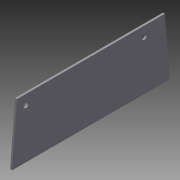
# Autodesk Inventor part: mountPiece
Saved by Autodesk Inventor 2015 SP1 (Build 190203100, 203)
## iProperties
Created: 2015-02-16
Part Number: mountPiece
Material: Generic
Document SubType Name: Modeling
Designer: 55221
Density: 1 g/cm^3
Appearance: Default
Author: 55221
Autodesk Inventor part; units mm, degrees
ref_plane "YZ Plane" through (0, 0, 0) normal (1, 0, 0) x (0, 1, 0)
ref_plane "XZ Plane" through (0, 0, 0) normal (0, 1, 0) x (-1, 0, 0)
ref_plane "XY Plane" through (0, 0, 0) normal (0, 0, 1) x (1, 0, 0)
sketch "Sketch1" plane through (0, 0, 0) normal (1, 0, 0) x (0, 1, 0)
  line L0 (50.8, 190.5) -> (0, 190.5)
  line L1 (0, 190.5) -> (0, 0)
  line L2 (0, 0) -> (50.8, 0)
  line L3 (50.8, 0) -> (50.8, 190.5)
  line L4 (0, 196.85) -> (50.8, 190.5)
  line L5 (0, 196.85) -> (0, 190.5)
  line L6 (0, 0) -> (50.8, 0)
  line L7 (0, 0) -> (0, 0)
  line L8 (50.8, 0) -> (0, 0)
  line L9 (0, 0) -> (0, 0)
  line L10 (0, -6.35) -> (50.8, 0)
  line L11 (0, -6.35) -> (0, 0)
  line L12 (0, 0) -> (76.2, 0)
  line L13 (76.2, 0) -> (76.2, 190.5)
  line L14 (76.2, 190.5) -> (0, 196.85)
  line L15 (76.2, 0) -> (0, -6.35)
  dimension "d0" = 76.2
  constraints: 32 end point, 4 perpendicular, 2 horizontal, 2 parallel, 1 collinear, 1 point on line, 1 vertical
  measures "d0" distance of L8.end L12.end
extrude "Extrusion1" add sketch "Sketch1" along normal blind 2.54
hole "Hole1" at (2.54, 63.5, 178.8143) direction (-1, 0, 0) diameter 6.35 end through all
pattern_linear "Rectangular Pattern1" count 2 spacing 152.4 along (0, 0, -1) of "Hole1"
body "Solid1"
